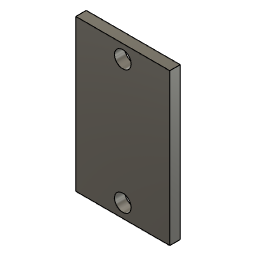
CP-BO Encoder locker v1 (Autodesk Fusion 360 design; units mm, degrees)
Autodesk Fusion 360 part; units mm, degrees
sketch "Esquisse1" plane through (0, 0, 0) normal (0, 0, 1) x (1, 0, 0)
  line L0 (0, 0) -> (18, 0)
  line L1 (18, 0) -> (18, 29)
  line L2 (18, 29) -> (0, 29)
  line L3 (0, 29) -> (0, 0)
  line L4 (9, 29) -> (9, 0) construction
  circle A0 centre (9, 26.4) radius 1.6
  circle A1 centre (9, 2.6) radius 1.6
  dimension "d1" = 18
  dimension "d2" = 29
  dimension "d3" = 3.2
  dimension "d4" = 3.2
  dimension "d5" = 2.6
  dimension "d6" = 2.6
  constraint horizontal L0
  constraint vertical L1
  constraint horizontal L2
  constraint vertical L3
  constraint coincident L0.start L3.end
  constraint midpoint L2 L4.start
  constraint midpoint L0 L4.end
  constraint coincident L4 A0.centre
  constraint coincident L4 A1.centre
  measures "d1" distance of L0.start L0.end
  measures "d2" distance of L0.start L2.end
  measures "d3" diameter of A0
  measures "d4" diameter of A1
  measures "d5" distance of L4.end A1.centre
  measures "d6" distance of L2 A0.centre
extrude "Extrusion1" add sketch "Esquisse1" along normal blind 2
